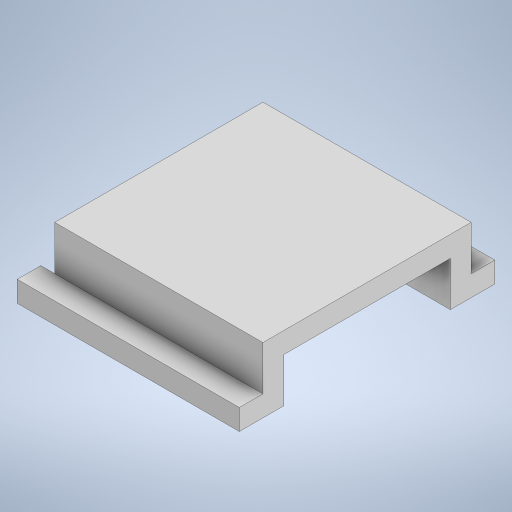
# Autodesk Inventor part: ZadBabkaPodkladka
Saved by Autodesk Inventor 2024 (Build 280153000, 153)
## iProperties
Created: 2023-11-13
Part Number: ZadBabkaPodkladka
Material: Generic
Document SubType Name: Modeling
Designer: KirikDK
Density: 1 g/cm^3
Appearance: Default
Author: KirikDK
Autodesk Inventor part; units mm, degrees
ref_plane "YZ Plane" through (0, 0, 0) normal (1, 0, 0) x (0, 1, 0)
ref_plane "XZ Plane" through (0, 0, 0) normal (0, 1, 0) x (-1, 0, 0)
ref_plane "XY Plane" through (0, 0, 0) normal (0, 0, 1) x (1, 0, 0)
sketch "Sketch1" plane through (0, 0, 0) normal (0, 1, 0) x (-1, 0, 0)
  line L0 (75, 33.3333) -> (-75, 33.3333)
  line L1 (-75, 33.3333) -> (-75, -116.6667)
  line L2 (-75, -116.6667) -> (75, -116.6667)
  line L3 (75, -116.6667) -> (75, 33.3333)
  point P0 (0, 0)
  dimension "d0" = 150
  dimension "d1" = 150
  constraints: 8 end point, 2 parallel, 1 horizontal, 1 perpendicular
  measures "d0" distance of L2.end L0.start
  measures "d1" distance of L0.start L0.end
extrude "Extrusion1" add sketch "Sketch1" along normal blind 47
sketch "Sketch2" plane through (75, 0, 33.3333) normal (1, 0, 0) x (0, 0, -1)
  line L0 (15, -11) -> (135, -11)
  line L1 (135, -11) -> (135, 32)
  line L2 (135, 32) -> (15, 32)
  line L3 (15, 32) -> (15, -11)
  line L4 (0, 47) -> (150, 47) projected
  line L5 (150, 0) -> (150, 47) projected
  line L6 (0, 0) -> (0, 47) projected
  point P0 (33.3333, 0)
  dimension "d4" = 15
  dimension "d5" = 15
  dimension "d6" = 15
  constraints: 8 end point, 2 parallel, 1 horizontal, 1 perpendicular
  measures "d4" distance between parallel lines of L4 L2
  measures "d5" distance between parallel lines of L5 L1
  measures "d6" distance between parallel lines of L6 L3
extrude "Extrusion2" cut sketch "Sketch2" against normal blind 200
sketch "Sketch3" plane through (75, 0, -116.6667) normal (1, 0, 0) x (0, 0, -1)
  line L0 (-150, 0) -> (-150, 47) projected
  line L1 (-150, 0) -> (-167, 0)
  line L2 (-167, 0) -> (-167, 15)
  line L3 (-167, 15) -> (-150, 15)
  line L4 (-150, 15) -> (-150, 0)
  line L5 (0, 0) -> (0, 47) projected
  line L6 (0, 0) -> (17, 0)
  line L7 (17, 0) -> (17, 15)
  line L8 (17, 15) -> (0, 15)
  line L9 (0, 15) -> (0, 0)
  point P0 (-116.6667, 0)
  point P1 (0, 15)
  dimension "d9" = 17
  dimension "d10" = 17
  dimension "d11" = 15
  dimension "d12" = 15
  constraints: 16 end point, 4 parallel, 2 horizontal, 2 perpendicular
  measures "d9" distance between parallel lines of L5 L7
  measures "d10" distance between parallel lines of L0 L2
  measures "d11" distance of L6.end L7.end
  measures "d12" distance of L1.end L2.end
extrude "Extrusion3" add sketch "Sketch3" against normal blind 160
body "Solid1"
